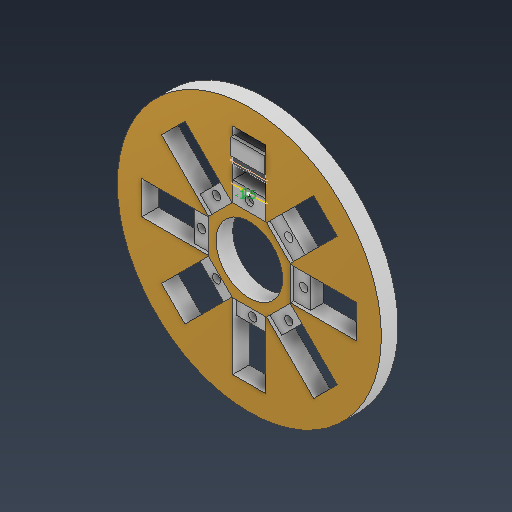
# Autodesk Inventor part: demo
Saved by Autodesk Inventor 2025.3 (Build 293356000, 356)
## iProperties
Created: 2025-12-15
Part Number: demo
Material: 一般
Document SubType Name: Modeling
Designer: 陳泓任
Density: 1 g/cm^3
Appearance: 預設
Author: 陳泓任
Autodesk Inventor part; units mm, degrees
ref_plane "YZ Plane" through (0, 0, 0) normal (1, 0, 0) x (0, 1, 0)
ref_plane "XZ Plane" through (0, 0, 0) normal (0, 1, 0) x (-1, 0, 0)
ref_plane "XY Plane" through (0, 0, 0) normal (0, 0, 1) x (1, 0, 0)
sketch "草圖1" plane through (0, 0, 0) normal (0, 0, 1) x (1, 0, 0)
  circle A0 centre (0, 0) radius 79.3187
  circle A1 centre (0, 0) radius 20
  line L0 (0, -92.0755) -> (0, 92.0755) construction
  circle A2 centre (0, 0) radius 54.6822 construction
  line L1 (-10, 49.6822) -> (10, 49.6822)
  line L2 (10, 49.6822) -> (10, 59.6822)
  line L3 (10, 59.6822) -> (-10, 59.6822)
  line L4 (-10, 59.6822) -> (-10, 49.6822)
  line L5 (-10, 49.6822) -> (10, 59.6822) construction
  line L6 (10, 49.6822) -> (-10, 59.6822) construction
  line L7 (10, 34.6822) -> (10, 64.6822)
  line L8 (10, 64.6822) -> (-10, 64.6822)
  line L9 (-10, 64.6822) -> (-10, 34.6822)
  line L10 (-10, 34.6822) -> (10, 34.6822)
  line L11 (10, 34.6822) -> (-10, 64.6822) construction
  line L12 (10, 64.6822) -> (-10, 34.6822) construction
  line L13 (-90.4266, 0) -> (90.4266, 0) construction
  line L14 (-38.6662, 52.8083) -> (-52.8083, 38.6662)
  line L15 (-52.8083, 38.6662) -> (-31.5951, 17.453)
  line L16 (-31.5951, 17.453) -> (-17.453, 31.5951)
  line L17 (-17.453, 31.5951) -> (-38.6662, 52.8083)
  line L18 (-64.6822, 10) -> (-64.6822, -10)
  line L19 (-64.6822, -10) -> (-34.6822, -10)
  line L20 (-34.6822, -10) -> (-34.6822, 10)
  line L21 (-34.6822, 10) -> (-64.6822, 10)
  line L22 (-52.8083, -38.6662) -> (-38.6662, -52.8083)
  line L23 (-38.6662, -52.8083) -> (-17.453, -31.5951)
  line L24 (-17.453, -31.5951) -> (-31.5951, -17.453)
  line L25 (-31.5951, -17.453) -> (-52.8083, -38.6662)
  line L26 (-10, -64.6822) -> (10, -64.6822)
  line L27 (10, -64.6822) -> (10, -34.6822)
  line L28 (10, -34.6822) -> (-10, -34.6822)
  line L29 (-10, -34.6822) -> (-10, -64.6822)
  line L30 (38.6662, -52.8083) -> (52.8083, -38.6662)
  line L31 (52.8083, -38.6662) -> (31.5951, -17.453)
  line L32 (31.5951, -17.453) -> (17.453, -31.5951)
  line L33 (17.453, -31.5951) -> (38.6662, -52.8083)
  line L34 (64.6822, -10) -> (64.6822, 10)
  line L35 (64.6822, 10) -> (34.6822, 10)
  line L36 (34.6822, 10) -> (34.6822, -10)
  line L37 (34.6822, -10) -> (64.6822, -10)
  line L38 (52.8083, 38.6662) -> (38.6662, 52.8083)
  line L39 (38.6662, 52.8083) -> (17.453, 31.5951)
  line L40 (17.453, 31.5951) -> (31.5951, 17.453)
  line L41 (31.5951, 17.453) -> (52.8083, 38.6662)
  line L42 (-28.0596, 42.2017) -> (-35.1307, 49.2728)
  line L43 (-49.2728, 35.1307) -> (-42.2017, 28.0596)
  line L44 (-35.1307, 49.2728) -> (-49.2728, 35.1307)
  line L45 (-42.2017, 28.0596) -> (-28.0596, 42.2017)
  line L46 (-49.6822, 10) -> (-59.6822, 10)
  line L47 (-59.6822, -10) -> (-49.6822, -10)
  line L48 (-59.6822, 10) -> (-59.6822, -10)
  line L49 (-49.6822, -10) -> (-49.6822, 10)
  line L50 (-42.2017, -28.0596) -> (-49.2728, -35.1307)
  line L51 (-35.1307, -49.2728) -> (-28.0596, -42.2017)
  line L52 (-49.2728, -35.1307) -> (-35.1307, -49.2728)
  line L53 (-28.0596, -42.2017) -> (-42.2017, -28.0596)
  line L54 (-10, -49.6822) -> (-10, -59.6822)
  line L55 (10, -59.6822) -> (10, -49.6822)
  line L56 (-10, -59.6822) -> (10, -59.6822)
  line L57 (10, -49.6822) -> (-10, -49.6822)
  line L58 (28.0596, -42.2017) -> (35.1307, -49.2728)
  line L59 (49.2728, -35.1307) -> (42.2017, -28.0596)
  line L60 (35.1307, -49.2728) -> (49.2728, -35.1307)
  line L61 (42.2017, -28.0596) -> (28.0596, -42.2017)
  line L62 (49.6822, -10) -> (59.6822, -10)
  line L63 (59.6822, 10) -> (49.6822, 10)
  line L64 (59.6822, -10) -> (59.6822, 10)
  line L65 (49.6822, 10) -> (49.6822, -10)
  line L66 (42.2017, 28.0596) -> (49.2728, 35.1307)
  line L67 (35.1307, 49.2728) -> (28.0596, 42.2017)
  line L68 (49.2728, 35.1307) -> (35.1307, 49.2728)
  line L69 (28.0596, 42.2017) -> (42.2017, 28.0596)
  circle A3 centre (0, 30.6822) radius 2.5
  line L70 (-10, 24.6822) -> (10, 24.6822) construction
  line L71 (10, 24.6822) -> (10, 36.6822) construction
  line L72 (10, 36.6822) -> (-10, 36.6822) construction
  line L73 (-10, 36.6822) -> (-10, 24.6822) construction
  line L74 (10, 36.6822) -> (-10, 24.6822) construction
  line L75 (-10, 36.6822) -> (10, 24.6822) construction
  circle A4 centre (-21.6956, 21.6956) radius 2.5
  circle A5 centre (-30.6822, 0) radius 2.5
  circle A6 centre (-21.6956, -21.6956) radius 2.5
  circle A7 centre (0, -30.6822) radius 2.5
  circle A8 centre (21.6956, -21.6956) radius 2.5
  circle A9 centre (30.6822, 0) radius 2.5
  circle A10 centre (21.6956, 21.6956) radius 2.5
  point P0 (0, 54.6822)
  point P1 (0, 49.6822)
  point P2 (0, 49.6822)
  dimension "d2" = 109.3645
  dimension "d0" = 40
  dimension "d1" = 158.6374
  dimension "d3" = 20
  dimension "d4" = 10
  dimension "d6" = 30
  dimension "d7" = 5
  dimension "d10" = 360
  dimension "d16" = 360
  dimension "d43" = 5
  dimension "d55" = 12
  dimension "d56" = 2
  dimension "d59" = 360
  constraints: 152 end point, 11 coincident, 10 centre point, 8 midpoint, 6 parallel, 3 horizontal, 3 perpendicular, 3 point on line, 2 collinear, 1 vertical, 1 vertical alignment, 157 other
  measures "d0" diameter of A1
  measures "d1" diameter of A0
  measures "d3" distance of L2.end L3.end
  measures "d4" distance of L1.end L2.end
  measures "d6" distance of L7.start L7.end
  measures "d7" distance of point (0, 49.682) point (0, 54.682)
  measures "d43" diameter of A3
  measures "d55" distance of L72.end L70.start
  measures "d56" distance between parallel lines of L10 L72
extrude "擠出1" add sketch "草圖1" along normal mid plane 10
sketch "草圖2" plane through (0, 0, 0) normal (0, 0, 1) x (1, 0, 0)
  line L0 (-10, 34.6822) -> (-10, 64.6822) construction
  line L1 (10, 64.6822) -> (10, 34.6822) construction
  line L2 (-10, 44.6822) -> (10, 44.6822)
  line L3 (10, 44.6822) -> (10, 59.6822)
  line L4 (10, 59.6822) -> (-10, 59.6822)
  line L5 (-10, 59.6822) -> (-10, 44.6822)
  line L6 (10, 59.6822) -> (-10, 59.6822) projected
  point P0 (0, 0)
  dimension "d50" = 15
  constraints: 8 end point, 2 parallel, 2 point on line, 1 collinear, 1 horizontal, 1 perpendicular
  measures "d50" distance between parallel lines of L4 L2
extrude "擠出2" add sketch "草圖2" along normal mid plane 7.9 separate body
sketch "草圖3" plane through (0, 0, 3.95) normal (0, 0, 1) x (1, 0, 0)
  line L0 (-10, 64.6822) -> (-10, 34.6822) construction
  line L1 (10, 34.6822) -> (10, 64.6822) construction
  line L2 (-10, 44.6822) -> (10, 44.6822)
  line L3 (10, 44.6822) -> (10, 49.6822)
  line L4 (10, 49.6822) -> (-10, 49.6822)
  line L5 (-10, 49.6822) -> (-10, 44.6822)
  line L6 (-10, 44.6822) -> (10, 44.6822) construction
  point P0 (0, 0)
  constraints: 8 end point, 2 parallel, 1 collinear, 1 horizontal, 1 midpoint, 1 perpendicular, 1 point on line
extrude "擠出3" add sketch "草圖3" along normal mid plane 2.1 bodies 2
sketch "草圖5" plane through (0, 0, 3.95) normal (0, 0, 1) x (1, 0, 0)
  line L0 (-10, 49.6822) -> (10, 49.6822) projected
  line L1 (10, 49.6822) -> (10, 59.6822) projected
  line L2 (10, 59.6822) -> (-10, 59.6822) projected
  line L3 (-10, 59.6822) -> (-10, 49.6822) projected
  point P0 (0, 0)
extrude "擠出6" add sketch "草圖5" along normal blind 2.1 separate body
sketch "草圖7" plane through (0, 0, 0) normal (1, 0, 0) x (0, 1, 0)
  line L0 (34.6822, 3) -> (34.6822, -5)
  line L1 (34.6822, 5) -> (44.6822, 5) construction
  line L2 (34.6822, -5) -> (34.6822, 5) projected
  line L3 (24.6822, 3) -> (24.6822, 5)
  line L4 (24.6822, 5) -> (36.6822, 5)
  line L5 (36.6822, -5) -> (34.6822, -5)
  arc A0 (38.6822, -1) -> (38.6822, 1) centre (38.6822, 0) ccw
  line L6 (38.6822, -1) -> (37.6822, -1)
  line L7 (38.6822, 1) -> (37.6822, 1)
  line L8 (36.6822, 5) -> (36.6822, 2)
  line L9 (36.6822, -2) -> (36.6822, -5)
  arc A1 (36.6822, 2) -> (37.6822, 1) centre (37.6822, 2) ccw
  arc A2 (37.6822, -1) -> (36.6822, -2) centre (37.6822, -2) ccw
  line L10 (34.6822, 0) -> (40.299, 0) construction
  line L11 (36.6822, -2) -> (36.6822, 2)
  line L12 (24.6822, 3) -> (34.6822, 3)
  point P0 (0, 0)
  dimension "d32" = 90
  dimension "d34" = 2
  dimension "d35" = 12
  dimension "d52" = 1
  dimension "d53" = 2
  dimension "d54" = 2
  dimension "d87" = 2
  constraints: 24 end point, 6 point on circle, 6 tangent, 4 horizontal, 4 perpendicular, 3 centre point, 3 collinear, 2 point on line, 2 vertical, 1 equal radius, 1 midpoint
  measures "d32" angle of L0 L1
  measures "d34" distance of L3.start L3.end
  measures "d35" distance of L3.end L4.end
  measures "d52" radius of A1
  measures "d53" diameter of A0
  measures "d54" distance from line of A0.centre L8
  measures "d87" distance between parallel lines of L0 L8
extrude "擠出7" add sketch "草圖7" along normal mid plane 20 separate body contours L2 L4 L8 L11 L9 L5 L0 | L12 L3 L4 L2
sketch "草圖16" plane through (0, 0, 5) normal (0, 0, 1) x (1, 0, 0)
  line L0 (10, 34.6822) -> (-10, 34.6822) projected
  line L1 (10, 24.6822) -> (10, 34.6822) projected
  line L2 (-10, 34.6822) -> (10, 34.6822)
  line L3 (10, 34.6822) -> (10, 24.6822)
  line L4 (10, 24.6822) -> (-10, 24.6822)
  line L5 (-10, 24.6822) -> (-10, 34.6822)
  line L6 (-31.5951, 17.453) -> (-17.453, 31.5951)
  line L7 (-17.453, 31.5951) -> (-10.3819, 24.524)
  line L8 (-10.3819, 24.524) -> (-24.524, 10.3819)
  line L9 (-24.524, 10.3819) -> (-31.5951, 17.453)
  line L10 (-34.6822, -10) -> (-34.6822, 10)
  line L11 (-34.6822, 10) -> (-24.6822, 10)
  line L12 (-24.6822, 10) -> (-24.6822, -10)
  line L13 (-24.6822, -10) -> (-34.6822, -10)
  line L14 (-17.453, -31.5951) -> (-31.5951, -17.453)
  line L15 (-31.5951, -17.453) -> (-24.524, -10.3819)
  line L16 (-24.524, -10.3819) -> (-10.3819, -24.524)
  line L17 (-10.3819, -24.524) -> (-17.453, -31.5951)
  line L18 (10, -34.6822) -> (-10, -34.6822)
  line L19 (-10, -34.6822) -> (-10, -24.6822)
  line L20 (-10, -24.6822) -> (10, -24.6822)
  line L21 (10, -24.6822) -> (10, -34.6822)
  line L22 (31.5951, -17.453) -> (17.453, -31.5951)
  line L23 (17.453, -31.5951) -> (10.3819, -24.524)
  line L24 (10.3819, -24.524) -> (24.524, -10.3819)
  line L25 (24.524, -10.3819) -> (31.5951, -17.453)
  line L26 (34.6822, 10) -> (34.6822, -10)
  line L27 (34.6822, -10) -> (24.6822, -10)
  line L28 (24.6822, -10) -> (24.6822, 10)
  line L29 (24.6822, 10) -> (34.6822, 10)
  line L30 (17.453, 31.5951) -> (31.5951, 17.453)
  line L31 (31.5951, 17.453) -> (24.524, 10.3819)
  line L32 (24.524, 10.3819) -> (10.3819, 24.524)
  line L33 (10.3819, 24.524) -> (17.453, 31.5951)
  point P0 (0, 0)
  dimension "d83" = 360
  constraints: 64 end point, 2 parallel, 1 horizontal, 1 perpendicular, 73 other
extrude "擠出9" cut sketch "草圖16" against normal blind 2 bodies 1
sketch "草圖8" plane through (-10, 24.6822, 5) normal (0, 0, 1) x (1, 0, 0)
  line L0 (10, -68.5126) -> (10, 19.1481) construction
  circle A0 centre (10, 6) radius 2.5
  line L1 (0, 10) -> (0, 40) construction
  line L2 (0, 12) -> (20, 12) construction
  line L3 (0, 0) -> (20, 0) construction
  line L4 (20, 12) -> (0, 0) construction
  line L5 (0, 12) -> (20, 0) construction
  point P0 (10, -24.6822)
  point P1 (10, 6)
  dimension "d39" = 5
  constraints: 6 end point, 3 midpoint, 1 centre point, 1 coincident, 1 vertical
  measures "d39" diameter of A0
extrude "擠出8" cut sketch "草圖8" against normal blind 20 bodies 4
ref_plane "工作平面2" through (-10, 34.6822, 3) normal (0, -1, 0) x (1, 0, 0)
sketch "草圖12" plane through (-10, 34.6822, 3) normal (0, -1, 0) x (1, 0, 0)
  line L0 (10, 2) -> (10, 3)
  line L1 (20, 0.95) -> (0, 0.95) projected
  line L2 (0, 2) -> (20, 2) projected
  arc A0 (10.75, 3) -> (9.25, 3) centre (10, 3) ccw
  line L3 (9.25, 3) -> (9.25, 2)
  line L4 (10.75, 3) -> (10.75, 2)
  point P0 (10, -3)
  dimension "d70" = 1
  dimension "d71" = 1.5
  constraints: 6 end point, 2 perpendicular, 2 point on circle, 2 point on line, 2 tangent, 1 centre point, 1 coincident, 1 midpoint, 1 vertical
  measures "d70" distance of L3.start L3.end
  measures "d71" diameter of A0
sketch "草圖13" plane through (-10, 24.6822, 5) normal (0, 0, 1) x (1, 0, 0)
  circle A0 centre (10.75, 10) radius 0.25
  point P0 (10, -24.6822)
  point P1 (10.75, 10)
  dimension "d72" = 0.5
  constraints: 1 centre point, 1 coincident
  measures "d72" diameter of A0
sweep "掃掠2" add profiles "草圖13" path "草圖12" bodies 4 path curves L4 A0 L3
ref_plane "工作平面3" through (-10, 46.6822, -3.95) normal (0, -1, 0) x (1, 0, 0)
sketch "草圖14" plane through (-10, 46.6822, -3.95) normal (0, -1, 0) x (1, 0, 0)
  line L0 (9.25, 8.95) -> (9.25, 9.95)
  line L1 (10.75, 8.95) -> (10.75, 9.95)
  arc A0 (10.75, 9.95) -> (9.25, 9.95) centre (10, 9.95) ccw
  line L2 (10, 8.5493) -> (10, 11.4408)
  line L3 (0, 8.95) -> (20, 8.95)
  point P0 (10, 3.95)
  point P1 (10, 8.95)
  dimension "d76" = 1
  dimension "d77" = 0.75
  constraints: 8 end point, 4 point on line, 3 vertical, 2 point on circle, 2 tangent, 1 centre point, 1 midpoint
  measures "d76" distance of L0.start L0.end
  measures "d77" radius of A0
sketch "草圖15" plane through (0, 0, 5) normal (0, 0, 1) x (1, 0, 0)
  circle A0 centre (0.75, 46.6822) radius 0.25
  point P0 (0, 0)
  dimension "d78" = 0.5
  constraints: 1 centre point, 1 coincident
  measures "d78" diameter of A0
sweep "掃掠3" add profiles "草圖15" path "草圖14" bodies 2 path curves L1 A0 L0
equation "\"d2\" = 2 * r_PM"
equation "\"d0\" = 2 * r_yi"
equation "\"d1\" = 2 * r_yo"
equation "\"d6\" = 3 * d4"
equation "\"d12\" = t_y"
equation "\"d19\" = t_y - t_PM"
equation "\"d21\" = t_PM"
equation "\"d30\" = t_PM"
equation "\"r_yo\" = 79.31871"
equation "\"r_PM\" = 54.68224"
equation "\"t_y\" = 10"
equation "\"t_PM\" = 2.1"
equation "\"w_PM\" = 38.6526"
equation "\"l_PM\" = 47.27293"
equation "\"PM_ratio\" = 0.9"
equation "\"r_yi\" = 20"
